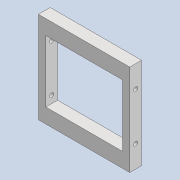
# Autodesk Inventor part: end_shell_n_1
Saved by Autodesk Inventor 2020 (Build 240168000, 168)
## iProperties
Created: 2021-10-06
Part Number: end_shell_n_1
Material: Generic
Document SubType Name: Modeling
Designer: Shuang Peng
Density: 1 g/cm^3
Appearance: Default
Author: Shuang Peng
Autodesk Inventor part; units mm, degrees
ref_plane "YZ Plane" through (0, 0, 0) normal (1, 0, 0) x (0, 1, 0)
ref_plane "XZ Plane" through (0, 0, 0) normal (0, 1, 0) x (-1, 0, 0)
ref_plane "XY Plane" through (0, 0, 0) normal (0, 0, 1) x (1, 0, 0)
sketch "Sketch1" plane through (0, 0, 0) normal (0, 0, 1) x (1, 0, 0)
  line L0 (-22, 14.1033) -> (-22, 5.8967) projected
  line L1 (2, 5.8967) -> (2, 14.1033) projected
  line L2 (-23, 0.5) -> (-23, 4) projected
  line L3 (-23, 16) -> (-23, 19.5) projected
  line L4 (3, 19.5) -> (3, 16) projected
  line L5 (3, 4) -> (3, 0.5) projected
  line L6 (2, 10) -> (-22, 10)
  line L7 (3, 20.5) -> (-23, 20.5)
  line L8 (-23, 20.5) -> (-23, -0.5)
  line L9 (-23, -0.5) -> (3, -0.5)
  line L10 (3, -0.5) -> (3, 20.5)
  line L11 (3, 20.5) -> (-23, -0.5) construction
  line L12 (-23, 20.5) -> (3, -0.5) construction
  line L13 (-20, 0.5) -> (-23, 0.5) projected
  line L14 (-20, 20) -> (-23, 20) projected
  line L15 (5.5, -5.5) -> (-25.5, -5.5)
  line L16 (-25.5, -5.5) -> (-25.5, 25.5)
  line L17 (-25.5, 25.5) -> (5.5, 25.5)
  line L18 (5.5, 25.5) -> (5.5, -5.5)
  line L19 (5.5, -5.5) -> (-25.5, 25.5) construction
  line L20 (-25.5, -5.5) -> (5.5, 25.5) construction
  point P0 (0, 0)
  point P1 (-10, 10)
  dimension "d0" = 26
  dimension "d1" = 21
  dimension "d2" = 5
  dimension "d3" = 2.5
  constraints: 26 end point, 7 midpoint, 4 parallel, 2 horizontal, 2 perpendicular
  measures "d0" distance of L9.end L8.end
  measures "d1" distance of L8.end L7.end
  measures "d2" distance between parallel lines of L17 L7
  measures "d3" distance between parallel lines of L16 L8
extrude "Extrusion1" add sketch "Sketch1" along normal mid plane 4
sketch "Sketch2" plane through (-25.5, -5.5, 2) normal (-1, 0, 0) x (0, 0, 1)
  circle A0 centre (-2, 23.5) radius 0.7 projected
  circle A1 centre (-2, 7.5) radius 0.7 projected
  point P0 (-2, 5.5)
extrude "Extrusion2" cut sketch "Sketch2" against normal up to surface (31 mm away)
body "Solid1"
